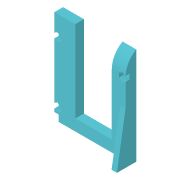
# Autodesk Inventor part: Back Wall with slant
Saved by Autodesk Inventor 2018 (Build 220112000, 112)
## iProperties
Created: 2018-12-27
Part Number: Back Wall with slant
Material: Generic
Document SubType Name: Modeling
Designer: ball
Density: 1 g/cm^3
Appearance: Default
Author: ball
Autodesk Inventor part; units mm, degrees
ref_plane "YZ Plane" through (0, 0, 0) normal (1, 0, 0) x (0, 1, 0)
ref_plane "XZ Plane" through (0, 0, 0) normal (0, 1, 0) x (-1, 0, 0)
ref_plane "XY Plane" through (0, 0, 0) normal (0, 0, 1) x (1, 0, 0)
ref_plane "Work Plane1" through (0, 0, 2.5241) normal (0, 0, 1) x (1, 0, 0)
sketch "Sketch1" plane through (0, 0, 2.5241) normal (0, 0, 1) x (1, 0, 0)
  line L0 (-4, 272) -> (-4, -8) construction
  line L1 (4, 272) -> (4, -8) construction
  line L2 (76, 272) -> (76, -8) construction
  line L3 (84, 272) -> (84, -8) construction
  line L4 (84, -8) -> (-4, -8) construction
  line L5 (84, 106) -> (80, 106) construction
  line L6 (80, 110) -> (76, 110) construction
  line L7 (-3.365, 272) -> (-3.365, -7.365) construction
  line L8 (-3.365, -7.365) -> (83.365, -7.365) construction
  line L9 (83.365, -7.365) -> (83.365, 272) construction
  line L10 (-3.365, -7.365) -> (83.365, -7.365)
  line L11 (83.365, -7.365) -> (83.365, 107.95)
  line L12 (-3.365, 107.95) -> (-3.365, -7.365)
  circle A0 centre (0, 12) radius 2
  circle A1 centre (80, 12) radius 2
  circle A2 centre (0, 84) radius 2
  circle A3 centre (80, 84) radius 2
  line L13 (21.39, 107.95) -> (21.39, 11.177)
  line L14 (21.39, 11.177) -> (67.11, 11.177)
  line L15 (67.11, 11.177) -> (67.11, 107.95)
  line L16 (83.365, 107.95) -> (67.11, 107.95)
  line L17 (21.39, 107.95) -> (-3.365, 107.95)
  point P0 (0, 0)
  dimension "d0" = 0.635
  dimension "d1" = 8.89
  dimension "d2" = 45.72
  dimension "d18" = 18.542
  constraints: 36 end point, 4 centre point, 4 horizontal, 4 parallel, 4 vertical, 1 perpendicular, 1 point on line, 22 other
  measures "d0" distance between parallel lines of L4 L8
  measures "d1" distance between parallel lines of L15 L2
  measures "d2" distance between parallel lines of L13 L15
  measures "d18" distance between parallel lines of L14 L8
extrude "Extrusion1" add sketch "Sketch1" along normal blind 10.16
sketch "Sketch2" plane through (0, 0, 12.6841) normal (0, 0, 1) x (1, 0, 0)
  line L0 (83.365, 107.95) -> (67.11, 107.95) projected
  line L1 (83.365, -7.365) -> (83.365, 107.95) projected
  line L2 (67.11, 107.95) -> (83.365, 107.95)
  line L3 (83.365, 107.95) -> (83.365, 23.8125)
  line L4 (67.11, 23.8125) -> (67.11, 107.95)
  circle A0 centre (80, 84) radius 2 projected
  circle A1 centre (80, 84) radius 1.9939
  line L5 (83.365, 23.8125) -> (83.365, -7.365)
  line L6 (83.365, -7.365) -> (67.11, -7.365)
  line L7 (67.11, -7.365) -> (67.11, 23.8125)
  point P0 (0, 0)
  dimension "d5" = 3.9878
  constraints: 12 end point, 2 parallel, 1 centre point, 1 coincident, 1 horizontal, 1 perpendicular, 1 point on line
  measures "d5" diameter of A1
extrude "Extrusion2" add sketch "Sketch2" along normal blind 2.54 contours L1 L6 L7 L4 L0
fillet "Fillet1" radius 25.4 1 edges at (75.2375, 107.95, 15.2241)
sketch "Sketch3" plane through (0, 0, 12.6841) normal (0, 0, 1) x (1, 0, 0)
  circle A0 centre (0, 12) radius 2 construction
  circle A1 centre (0, 12) radius 4.8768 construction
  circle A2 centre (0, 84) radius 2 construction
  circle A3 centre (0, 84) radius 4.8768 construction
  circle A4 centre (80, 12) radius 2 construction
  line L0 (0, 16.8768) -> (4.2234, 14.4384)
  line L1 (4.2234, 14.4384) -> (4.2234, 9.5616)
  line L2 (4.2234, 9.5616) -> (0, 7.1232)
  line L3 (0, 7.1232) -> (-4.2234, 9.5616)
  line L4 (-4.2234, 9.5616) -> (-4.2234, 14.4384)
  line L5 (-4.2234, 14.4384) -> (0, 16.8768)
  line L6 (0, 88.8768) -> (4.2234, 86.4384)
  line L7 (4.2234, 86.4384) -> (4.2234, 81.5616)
  line L8 (4.2234, 81.5616) -> (0, 79.1232)
  line L9 (0, 79.1232) -> (-4.2234, 81.5616)
  line L10 (-4.2234, 81.5616) -> (-4.2234, 86.4384)
  line L11 (-4.2234, 86.4384) -> (0, 88.8768)
  point P0 (0, 0)
  dimension "d9" = 9.7536
  dimension "d10" = 9.7536
  constraints: 24 end point, 5 coincident, 2 vertical alignment, 30 other
extrude "Extrusion3" cut sketch "Sketch3" against normal blind 4.826
sketch "Sketch4" plane through (0, 0, 15.2241) normal (0, 0, 1) x (1, 0, 0)
  circle A0 centre (80, 84) radius 2 construction
  circle A1 centre (80, 84) radius 4.8768 construction
  line L0 (80, 88.8768) -> (84.2234, 86.4384)
  line L1 (84.2234, 86.4384) -> (84.2234, 81.5616)
  line L2 (84.2234, 81.5616) -> (80, 79.1232)
  line L3 (80, 79.1232) -> (75.7766, 81.5616)
  line L4 (75.7766, 81.5616) -> (75.7766, 86.4384)
  line L5 (75.7766, 86.4384) -> (80, 88.8768)
  point P0 (0, 0)
  dimension "d14" = 9.7536
  constraints: 12 end point, 2 coincident, 1 vertical alignment, 15 other
extrude "Extrusion4" cut sketch "Sketch4" against normal blind 4.826
sketch "Sketch5" plane through (0, 0, 12.6841) normal (0, 0, 1) x (1, 0, 0)
  line L0 (-3.365, -7.365) -> (67.11, -7.365) projected
  line L1 (-3.365, -7.365) -> (67.11, -7.365)
  line L2 (67.11, 5.335) -> (-3.365, 5.335)
  line L3 (-3.365, 5.335) -> (-3.365, -7.365)
  line L4 (67.11, 5.335) -> (67.11, -7.365)
  line L5 (-3.365, -7.365) -> (83.365, -7.365) projected
  point P0 (0, 0)
  constraints: 8 end point, 1 horizontal, 1 parallel, 1 perpendicular, 1 point on line
extrude "Extrusion5" cut sketch "Sketch5" against normal blind 5.08
sketch "Sketch13" plane through (83.365, -7.365, 15.2241) normal (1, 0, 0) x (0, 0, -1)
  line L0 (0, 0) -> (7.62, 0) projected
  line L1 (0, 0) -> (-10.16, 0)
  line L2 (0, 93.318) -> (0, 0) projected
  line L3 (0, 0) -> (0, 60.96)
  line L4 (0, 60.96) -> (-10.16, 0)
  point P0 (15.2241, 7.365)
  dimension "d54" = 10.16
  dimension "d55" = 60.96
  constraints: 6 end point, 1 horizontal, 1 point on line
  measures "d54" distance of L0.start L1.end
  measures "d55" distance of L0.start L3.end
extrude "Extrusion13" add sketch "Sketch13" against normal blind 6.35
sketch "Sketch14" plane through (0, 0, 15.2241) normal (0, 0, 1) x (1, 0, 0)
  line L0 (67.11, -7.365) -> (77.015, -7.365) projected
  line L1 (77.015, -7.365) -> (77.015, 53.595) projected
  line L2 (67.11, -7.365) -> (77.015, -7.365)
  line L3 (77.015, -7.365) -> (77.015, 5.3272)
  line L4 (77.015, 5.3272) -> (67.11, 5.3272)
  line L5 (67.11, 5.3272) -> (67.11, -7.365)
  point P0 (0, 0)
  constraints: 8 end point, 2 parallel, 1 horizontal, 1 perpendicular, 1 point on line
extrude "Extrusion14" cut sketch "Sketch14" against normal up to surface (7.62 mm away)
body "Solid1"
